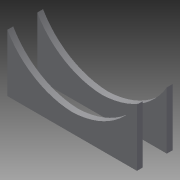
# Autodesk Inventor part: Robotics ball launcher guide
Saved by Autodesk Inventor 2014 (Build 180170000, 170)
## iProperties
Created: 2016-01-22
Part Number: Robotics ball launcher guide
Material: Generic
Document SubType Name: Modeling
Designer: shawnsargent
Density: 1 g/cm^3
Appearance: Default
Author: shawnsargent
Autodesk Inventor part; units mm, degrees
ref_plane "YZ Plane" through (0, 0, 0) normal (1, 0, 0) x (0, 1, 0)
ref_plane "XZ Plane" through (0, 0, 0) normal (0, 1, 0) x (-1, 0, 0)
ref_plane "XY Plane" through (0, 0, 0) normal (0, 0, 1) x (1, 0, 0)
sketch "Sketch1" plane through (0, 0, 0) normal (0, 0, 1) x (1, 0, 0)
  line L0 (0, 0) -> (445.0334, 0)
  line L1 (445.0334, 0) -> (445.0334, 196.85)
  line L2 (0, 0) -> (0, 196.85)
  arc A0 (0, 196.85) -> (222.5167, 63.5) centre (231.0477, 330.0635) ccw
  arc A1 (222.5167, 63.5) -> (445.0334, 196.85) centre (213.9857, 330.0635) ccw
  dimension "d0" = 445.0334
  dimension "d1" = 196.85
  dimension "d3" = 266.7
  dimension "d4" = 266.7
  constraints: 6 end point, 4 point on circle, 2 centre point, 1 horizontal, 1 parallel, 1 perpendicular
  measures "d0" distance of L0.start L0.end
  measures "d1" distance of L0.end L1.end
  measures "d3" radius of A0
  measures "d4" radius of A1
extrude "Extrusion1" add sketch "Sketch1" along normal blind 20.193
sketch "Sketch2" plane through (0, 0, 20.193) normal (0, 0, 1) x (1, 0, 0)
  line L0 (0, 0) -> (445.0334, 0) projected
  line L1 (111.2011, 0) -> (141.5914, 0)
  line L2 (141.5914, 0) -> (141.5914, 15.1977)
  line L3 (141.5914, 15.1977) -> (111.2011, 15.1977)
  line L4 (111.2011, 15.1977) -> (111.2011, 0)
  constraints: 8 end point, 2 parallel, 1 horizontal, 1 perpendicular, 1 point on line
extrude "Extrusion2" add sketch "Sketch2" along normal blind 82.3443
sketch "Sketch3" plane through (0, 0, 102.5373) normal (0, 0, 1) x (1, 0, 0)
  line L0 (111.2011, 0) -> (141.5914, 0) projected
  line L1 (141.5914, 0) -> (141.5914, 15.1977) projected
  line L2 (141.5914, 15.1977) -> (111.2011, 15.1977) projected
  line L3 (111.2011, 15.1977) -> (111.2011, 0) projected
  line L4 (141.5914, 15.1977) -> (141.5914, 0) projected
  line L5 (141.5914, 0) -> (445.0334, 0) projected
  line L6 (445.0334, 0) -> (445.0334, 196.85) projected
  arc A0 (222.5167, 63.5) -> (445.0334, 196.85) centre (213.9857, 330.0635) ccw projected
  arc A1 (0, 196.85) -> (222.5167, 63.5) centre (231.0477, 330.0635) ccw projected
  line L7 (0, 196.85) -> (0, 0) projected
  line L8 (0, 0) -> (111.2011, 0) projected
  line L9 (111.2011, 0) -> (111.2011, 15.1977) projected
  line L10 (111.2011, 15.1977) -> (141.5914, 15.1977) projected
extrude "Extrusion3" add sketch "Sketch3" along normal blind 20.193
sketch "Sketch4" plane through (111.2011, 15.1977, 20.193) normal (0, 1, 0) x (1, 0, 0)
  line L0 (0, 0) -> (30.3903, 0) projected
  line L1 (0, 0) -> (0, -82.3443) projected
  line L2 (30.3903, -82.3443) -> (0, -82.3443) projected
  line L3 (30.3903, 0) -> (30.3903, -82.3443) projected
  point P0 (-111.2011, 20.193)
extrude "Extrusion4" cut sketch "Sketch4" against normal blind 20.193
body "Solid1"
